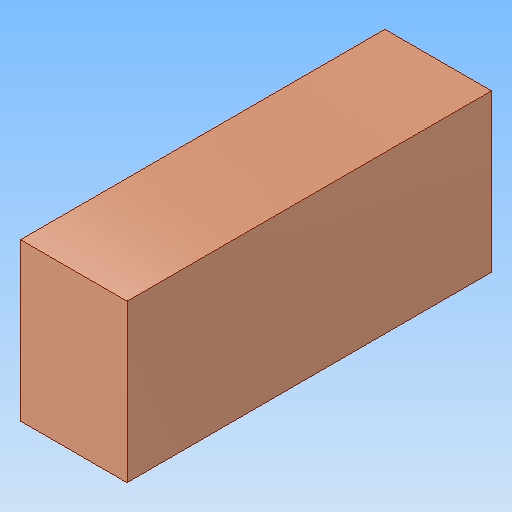
# Autodesk Inventor part: Деталь1
Saved by Autodesk Inventor 2019 (Build 230136000, 136)
## iProperties
Created: 2021-02-11
Part Number: Деталь1
Material: Дерево (дуб)
Document SubType Name: Modeling
Designer: Kurbatova
Density: 0.76 g/cm^3
Appearance: Белый дуб — натуральный — с умеренным глянцем
Author: Kurbatova
Autodesk Inventor part; units mm, degrees
ref_plane "YZ Plane" through (0, 0, 0) normal (1, 0, 0) x (0, 1, 0)
ref_plane "XZ Plane" through (0, 0, 0) normal (0, 1, 0) x (-1, 0, 0)
ref_plane "XY Plane" through (0, 0, 0) normal (0, 0, 1) x (1, 0, 0)
sketch "Эскиз1" plane through (0, 0, 0) normal (0, 0, 1) x (1, 0, 0)
  line L0 (-14.6366, 33.3503) -> (8555.5591, 33.3503)
  line L1 (8555.5591, 33.3503) -> (8555.5591, -12606.4104)
  line L2 (8555.5591, -12606.4104) -> (-14.6366, -12606.4104)
  line L3 (-14.6366, -12606.4104) -> (-14.6366, 33.3503)
  point P0 (0, 0)
  constraints: 8 end point, 2 parallel, 1 horizontal, 1 perpendicular
extrude "Выдавливание1" add sketch "Эскиз1" against normal blind 29311.5
